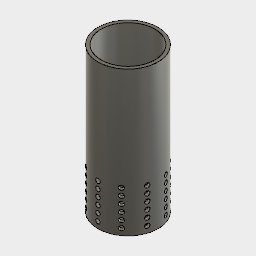
Case_Base (Autodesk Fusion 360 design; units mm, degrees)
Autodesk Fusion 360 part; units mm, degrees
sketch "Sketch1" plane through (0, 0, 0) normal (0, 1, 0) x (1, 0, 0)
  circle A0 centre (0, 0) radius 13.75
  dimension "d1" = 27.5
  measures "d1" diameter of A0
extrude "Extrude1" add sketch "Sketch1" along normal blind 66
sketch "Sketch2" plane through (0, 66, 0) normal (0, 1, 0) x (-1, 0, 0)
  circle A0 centre (0, 0) radius 13.75
  circle A1 centre (0, 0) radius 12.25
  dimension "d4" = 24.5
  measures "d4" diameter of A1
extrude "Extrude2" cut sketch "Sketch2" against normal blind 65 contours A1
ref_plane "WorkPlane1" through (0, 33, 13.75) normal (0, 0, 1) x (1, 0, 0)
sketch "Sketch4" plane through (0, 33, 13.75) normal (0, 0, 1) x (1, 0, 0)
  circle A0 centre (0, -30) radius 1
  line L0 (13.75, -33) -> (-13.75, -33)
  circle A1 centre (0, -26.8) radius 1
  circle A2 centre (0, -23.6) radius 1
  circle A3 centre (0, -20.4) radius 1
  circle A4 centre (0, -17.2) radius 1
  circle A5 centre (0, -14) radius 1
  dimension "d11" = 2
  dimension "d12" = 3
  dimension "d15" = 0
  dimension "d16" = 16
  measures "d11" diameter of A0
  measures "d12" distance of A0.centre L0
extrude "Extrude4" cut sketch "Sketch4" against normal through all
pattern_circular "C-Pattern1" count 5 over 360 about axis through (0, 1.75, 0) along (0, 1, 0) of "Extrude4"
